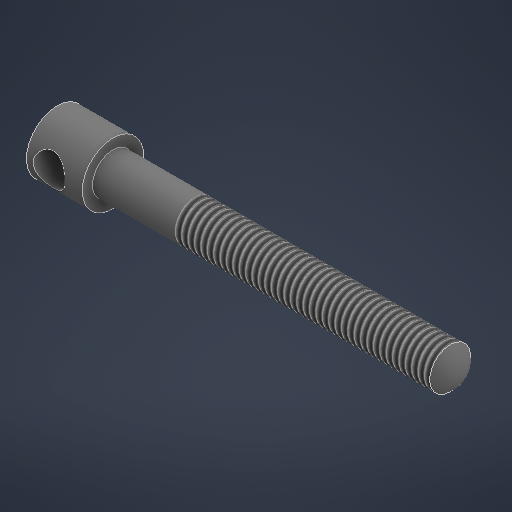
# Autodesk Inventor part: Mozgatóorsó
Saved by Autodesk Inventor 2025 (Build 290162010, 162A)
## iProperties
Created: 2025-02-13
Part Number: Mozgatóorsó
Material: Generic
Document SubType Name: Modeling
Designer: petruska.milan
Density: 1 g/cm^3
Appearance: Gray
Author: petruska.milan
Autodesk Inventor part; units mm, degrees
ref_plane "YZ Plane" through (0, 0, 0) normal (1, 0, 0) x (0, 1, 0)
ref_plane "XZ Plane" through (0, 0, 0) normal (0, 1, 0) x (-1, 0, 0)
sketch "Sketch1" plane through (0, 0, 0) normal (0, 0, 1) x (1, 0, 0)
  line L0 (0, 0) -> (80, 0)
  line L1 (80, 0) -> (80, 4)
  line L2 (80, 4) -> (0, 4)
  line L3 (0, 4) -> (0, 0)
  line L4 (80, 0) -> (75, 0)
  circle A0 centre (75, 0) radius 5
  line L5 (0, 0) -> (12, 0)
  line L6 (12, 0) -> (12, 6)
  line L7 (12, 6) -> (0, 6)
  line L8 (0, 6) -> (0, 0)
  line L9 (0, 0) -> (17, 0)
  circle A1 centre (17, 0) radius 17
  point P0 (78, 4)
  point P1 (12, 4)
  point P2 (1.094, 6)
  dimension "d0" = 80
  dimension "d1" = 4
  dimension "d2" = 5
  dimension "d3" = 12
  dimension "d4" = 6
  dimension "d5" = 17
  constraints: 20 end point, 4 parallel, 2 coincident, 2 horizontal, 2 perpendicular, 2 point on line, 6 other
  measures "d0" distance of L2.end L1.end
  measures "d1" distance of L1.end L0.end
  measures "d2" distance of L0.end L4.end
  measures "d3" distance of L7.end L6.end
  measures "d4" distance of L6.end L5.end
  measures "d5" distance of L0.start L9.end
revolve "Revolution1" add sketch "Sketch1" angle 360 about axis through (0, 0, 0) along (1, 0, 0) picked at (8.3647, 5.3333) contours A1 L2 L6 L0 | L6 L2 A1 L0 | A1 L2 A0 L0 | A1 L7 L6 L2 | A0 L2 L0
ref_plane "Work Plane1" through (6.547, 0, 6) normal (0, 0, 1) x (1, 0, 0)
sketch "Sketch2" plane through (6.547, 0, 6) normal (0, 0, 1) x (1, 0, 0)
  line L0 (5.453, -4) -> (5.453, 4) projected
  line L1 (5.453, 0) -> (-1.047, 0)
  circle A0 centre (-1.047, 0) radius 3.1
  point P0 (-6.547, 0)
  dimension "d7" = 6.5
  dimension "d8" = 6.2
  constraints: 2 end point, 1 centre point, 1 coincident, 1 horizontal, 1 midpoint
  measures "d7" distance of L1.start L1.end
  measures "d8" diameter of A0
extrude "Extrusion1" cut sketch "Sketch2" against normal through all
thread "Thread1" size "M8x1.25" class "6g" standard "ANSI Metric M Profile" length 50
body "Solid1"
